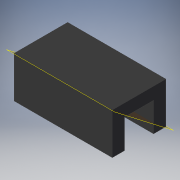
# Autodesk Inventor part: HookBracket2
Saved by Autodesk Inventor 2018 (Build 220112000, 112)
## iProperties
Created: 2019-05-03
Part Number: HookBracket2
Material: Generic
Document SubType Name: Modeling
Designer: anirudh
Density: 1 g/cm^3
Appearance: Default
Author: anirudh
Autodesk Inventor part; units mm, degrees
ref_plane "YZ Plane" through (0, 0, 0) normal (1, 0, 0) x (0, 1, 0)
ref_plane "XZ Plane" through (0, 0, 0) normal (0, 1, 0) x (-1, 0, 0)
ref_plane "XY Plane" through (0, 0, 0) normal (0, 0, 1) x (1, 0, 0)
sketch "Sketch10" plane through (0, 0, 0) normal (0, 1, 0) x (-1, 0, 0)
  line L0 (0, 0) -> (50.8, 0)
  line L1 (50.8, 0) -> (50.8, -15)
  line L2 (50.8, -15) -> (0, -15)
  line L3 (0, -15) -> (0, 0)
  dimension "d26" = 50.8
  dimension "d27" = 15
  constraints: 8 end point, 2 parallel, 1 horizontal, 1 perpendicular
  measures "d26" distance of L1.end L2.end
  measures "d27" distance of L0.end L1.end
extrude "Extrusion8" add sketch "Sketch10" along normal blind 6.35
sketch "Sketch11" plane through (0, 0, 0) normal (1, 0, 0) x (0, 0, -1)
  line L0 (0, 6.35) -> (-6.35, 6.35)
  line L1 (-6.35, 6.35) -> (-6.35, -15.0114)
  line L2 (-6.35, -15.0114) -> (0, -15.0114)
  line L3 (0, -15.0114) -> (0, 6.35)
  line L4 (15, 0) -> (15, 6.35) projected
  line L5 (15, 6.35) -> (21.35, 6.35)
  line L6 (21.35, 6.35) -> (21.35, -15.0114)
  line L7 (21.35, -15.0114) -> (15, -15.0114)
  line L8 (15, -15.0114) -> (15, 6.35)
  point P0 (0, 0)
  dimension "d30" = 6.35
  dimension "d31" = 21.3614
  dimension "d32" = 6.35
  constraints: 16 end point, 4 parallel, 2 horizontal, 2 perpendicular, 1 point on line
  measures "d30" distance of L2.end L1.end
  measures "d31" distance of L1.end L0.end
  measures "d32" distance of L6.end L7.end
extrude "Extrusion9" add sketch "Sketch11" against normal blind 50.8
ref_plane "Work Plane7" through (0, -15.0114, -21.35) normal (0, 0.7918814, -0.6106749) x (-1, 0, 0)
body "Solid2"
